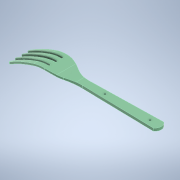
# Autodesk Inventor part: fork
Saved by Autodesk Inventor 2022 (Build 260153000, 153)
## iProperties
Created: 2022-10-22
Part Number: fork
Material: ポリスチレン
Document SubType Name: Modeling
Designer: Yazawa
Density: 1.021 g/cm^3
Appearance: 滑らか - 濃い海緑
Mass: 5.29286 g
Surface Area: 61.1423 cm^2
Volume: 5.18399 cm^3
Author: Yazawa
Autodesk Inventor part; units mm, degrees
ref_plane "YZ Plane" through (0, 0, 0) normal (1, 0, 0) x (0, 1, 0)
ref_plane "XY Plane" through (0, 0, 0) normal (0, 0, 1) x (1, 0, 0)
sketch "スケッチ2" plane through (0, 0, 0) normal (0, 0, 1) x (1, 0, 0)
  arc A0 (-71.334, 3.9069) -> (-94.9642, 3.9069) centre (-83.1491, -32.8019) ccw
  arc A1 (-71.334, 3.9069) -> (-56, 1.5) centre (-56, 51.5486) ccw
  arc A2 (-94.9642, 3.9069) -> (-123.954, -9.7731) centre (-56.9435, -114.2212) ccw
  line L0 (-56, 1.5) -> (34, 1.5)
  arc A3 (-71.9467, 2.0031) -> (-94.3514, 2.0031) centre (-83.1491, -32.8019) ccw
  arc A4 (-94.3514, 2.0031) -> (-122.874, -11.4564) centre (-56.9435, -114.2212) ccw
  line L1 (34, -1.5) -> (-49.6292, -1.5)
  arc A5 (-71.9467, 2.0031) -> (-49.6292, -1.5) centre (-49.6292, 71.3424) ccw
  line L2 (34, 1.5) -> (34, -1.5)
  line L3 (-123.954, -9.7731) -> (-122.874, -11.4564)
  line L4 (-71.9467, 2.0031) -> (-71.334, 3.9069) construction
  point P0 (0, 0)
  point P1 (-83.1491, 5.7615)
  point P2 (0, 0)
  point P3 (34, 0)
  dimension "d19" = 90
  dimension "d27" = 38.5634
  dimension "d28" = 124.096
  dimension "d29" = 14.842
  dimension "d49" = 50.0486
  dimension "d51" = 3
  dimension "d52" = 35.683
  dimension "d53" = 2
  dimension "d54" = 34
  constraints: 13 point on circle, 10 end point, 6 centre point, 5 tangent, 1 coincident, 1 horizontal, 1 horizontal alignment, 1 line through centre, 1 midpoint, 1 point on line, 1 vertical, 1 vertical alignment, 1 other
  measures "d19" distance of L0.start L0.end
  measures "d27" radius of A0
  measures "d28" radius of A2
  measures "d49" radius of A1
  measures "d51" distance between parallel lines of L0 L1
  measures "d53" distance of L3.start L3.end
  measures "d54" distance from line of L2 point (0, 0)
extrude "押し出し2" add sketch "スケッチ2" along normal mid plane 25.5
ref_plane "作業平面3" through (0, -15, 0) normal (0, 1, 0) x (-1, 0, 0)
sketch "スケッチ7" plane through (0, -15, 0) normal (0, 1, 0) x (-1, 0, 0)
  line L0 (-34, -12.75) -> (-34, 12.75) projected
  line L1 (-31, 5.8) -> (49.6292, 4.05)
  line L2 (49.6292, -4.05) -> (-31, -5.8)
  arc A0 (-31, 5.8) -> (-31, -5.8) centre (-26.8933, 0) ccw
  line L3 (49.6292, 4.05) -> (49.6292, -4.05)
  line L4 (49.6292, -12.75) -> (49.6292, 12.75) projected
  arc A1 (49.6292, 4.05) -> (66.3891, 8.3029) centre (50.332, 36.4306) ccw
  arc A2 (83.1491, 12.75) -> (66.3891, 8.3029) centre (83.1491, -21.0558) ccw
  arc A3 (123.023, 11.3723) -> (83.1491, 12.75) centre (83.1491, -564.9559) ccw
  line L5 (71.9467, 12.75) -> (94.3514, 12.75) projected
  line L6 (83.1491, 22.835) -> (66.3891, 22.835)
  line L7 (66.3891, 22.835) -> (49.6292, 22.835)
  line L8 (134.4168, 12.75) -> (134.4168, 6.375)
  line L9 (134.4168, 6.375) -> (134.4168, 0)
  line L10 (134.4168, 0) -> (134.4168, -6.375)
  line L11 (134.4168, -6.375) -> (134.4168, -12.75)
  line L12 (94.3514, -12.75) -> (71.9467, -12.75) projected
  arc A4 (123.023, 9.3771) -> (123.023, 11.3723) centre (122.954, 10.3747) ccw
  line L13 (122.954, 10.3747) -> (110.8745, 10.3747)
  arc A5 (83.1491, 7.9993) -> (123.023, 9.3771) centre (83.1491, 585.7052) ccw
  arc A6 (83.1491, 7.9993) -> (82.1491, 6.9993) centre (83.1491, 6.9993) ccw
  line L14 (123.954, -12.75) -> (123.954, 12.75) projected
  line L15 (83.1491, 6.9993) -> (89.0198, 6.9993)
  arc A7 (123.023, 2.6264) -> (123.023, 4.6216) centre (122.954, 3.624) ccw
  line L16 (122.954, 3.624) -> (110.8745, 3.624)
  arc A8 (123.023, 4.6216) -> (83.1491, 5.9993) centre (83.1491, -571.7065) ccw
  arc A9 (82.1491, 6.9993) -> (83.1491, 5.9993) centre (83.1491, 6.9993) ccw
  arc A10 (83.1491, 1.2487) -> (123.023, 2.6264) centre (83.1491, 578.9546) ccw
  arc A11 (83.1491, 1.2487) -> (81.9004, 0) centre (83.1491, 0) ccw
  line L17 (83.1491, 0) -> (89.0198, 0)
  arc A12 (83.1491, -12.75) -> (123.023, -11.3723) centre (83.1491, 564.9559) ccw
  arc A13 (123.023, -11.3723) -> (123.023, -9.3771) centre (122.954, -10.3747) ccw
  arc A14 (123.023, -9.3771) -> (83.1491, -7.9993) centre (83.1491, -585.7052) ccw
  arc A15 (82.1491, -6.9993) -> (83.1491, -7.9993) centre (83.1491, -6.9993) ccw
  arc A16 (123.023, -4.6216) -> (123.023, -2.6264) centre (122.954, -3.624) ccw
  arc A17 (83.1491, -5.9993) -> (123.023, -4.6216) centre (83.1491, 571.7065) ccw
  arc A18 (83.1491, -5.9993) -> (82.1491, -6.9993) centre (83.1491, -6.9993) ccw
  arc A19 (123.023, -2.6264) -> (83.1491, -1.2487) centre (83.1491, -578.9546) ccw
  arc A20 (81.9004, 0) -> (83.1491, -1.2487) centre (83.1491, 0) ccw
  arc A21 (66.3891, -8.3029) -> (49.6292, -4.05) centre (50.332, -36.4306) ccw
  arc A22 (66.3891, -8.3029) -> (83.1491, -12.75) centre (83.1491, 21.0558) ccw
  point P0 (-34, 0)
  point P1 (-34, 0)
  point P2 (49.6292, 0)
  point P3 (134.4168, 9.5625)
  point P4 (134.4168, 3.1875)
  point P5 (134.4168, -3.1875)
  point P6 (134.4168, -9.5625)
  dimension "d60" = 8.1
  dimension "d61" = 11.6
  dimension "d62" = 3
  dimension "d67" = 1
  dimension "d68" = 1
  constraints: 56 point on circle, 32 symmetric about line, 26 end point, 23 centre point, 8 midpoint, 8 tangent, 5 coincident, 5 point on line, 5 vertical alignment, 4 collinear, 3 horizontal, 3 vertical, 1 horizontal alignment, 16 other
  measures "d60" distance of L1.end L2.start
  measures "d61" distance of L2.end L1.start
  measures "d62" horizontal distance of point (-34, 0) L1.start
  measures "d67" radius of A4
  measures "d68" radius of A6
extrude "押し出し4" cut sketch "スケッチ7" along normal blind 25.5 contours L1 L3 L2 A0 | A1 A2 A3 A4 A5 A6 A9 A8 A7 A10 A11 A20 A19 A16 A17 A18 A15 A14 A13 A12 A22 A21 L3 keep common part
sketch "スケッチ8" plane through (0, -15, 0) normal (0, 1, 0) x (-1, 0, 0)
  arc A0 (-31, 5.8) -> (-31, -5.8) centre (-26.8933, 0) ccw projected
  point P0 (0, 0)
  point P1 (-21.5, 0)
  point P2 (28.5, 0)
  point P3 (-34, 0)
  dimension "d71" = 50
  dimension "d72" = 12.5
  constraints: 3 horizontal alignment, 1 point on circle
  measures "d71" distance of point (-21.5, 0) point (28.5, 0)
  measures "d72" distance of point (-21.5, 0) point (-34, 0)
hole "穴2" at (21.5, -15, 0) at (-28.5, -15, 0) direction (0, 1, 0) diameter 2.459 end through all thread size "M3x0.5" class "6H" standard "ISO Metric profile"
